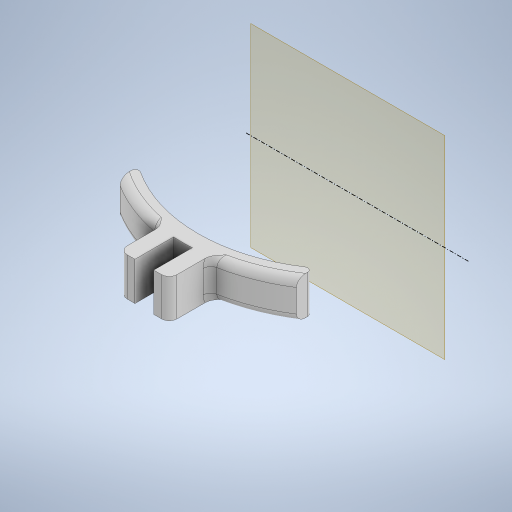
# Autodesk Inventor part: 날개꼽는파트
Saved by Autodesk Inventor 2023 (Build 270158000, 158)
## iProperties
Created: 2023-08-28
Part Number: 날개꼽는파트
Material: 일반
Document SubType Name: Modeling
Designer: rlatk
Density: 1 g/cm^3
Appearance: 기본값
Author: rlatk
Autodesk Inventor part; units mm, degrees
ref_plane "YZ Plane" through (0, 0, 0) normal (1, 0, 0) x (0, 1, 0)
ref_plane "XZ Plane" through (0, 0, 0) normal (0, 1, 0) x (-1, 0, 0)
sketch "스케치1" plane through (0, 0, 0) normal (0, 1, 0) x (-1, 0, 0)
  line L0 (-6.5, -10) -> (-6.5, 10)
  line L1 (6.5, 10) -> (6.5, -10)
  line L2 (6.5, -10) -> (-6.5, 10) construction
  line L3 (-6.5, -10) -> (6.5, 10) construction
  line L4 (2.45, -10) -> (-2.45, -10)
  line L5 (-2.45, -10) -> (-2.45, 10)
  line L6 (-2.45, 10) -> (2.45, 10)
  line L7 (2.45, 10) -> (2.45, -10)
  line L8 (2.45, -10) -> (-2.45, 10) construction
  line L9 (-2.45, -10) -> (2.45, 10) construction
  arc A0 (22.9827, -6.6573) -> (-22.9827, -6.6573) centre (0, -43) ccw
  arc A1 (22.9827, -11.4914) -> (-22.9827, -11.4914) centre (0, -43) ccw
  line L10 (22.9827, -11.4914) -> (22.9827, -6.6573)
  line L11 (-22.9827, -11.4914) -> (-22.9827, -6.6573)
  line L12 (-6.5, 10) -> (-2.45, 10)
  line L13 (2.45, 10) -> (6.5, 10)
  line L14 (6.5, -10) -> (2.45, -10)
  line L15 (-2.45, -10) -> (-6.5, -10)
  point P0 (0, 0)
  point P1 (6.5, -0.4941)
  point P2 (2.45, -0.0699)
  point P3 (-2.45, -0.0699)
  point P4 (-6.5, -0.4941)
  dimension "d0" = 13
  dimension "d1" = 20
  dimension "d2" = 4.9
  dimension "d3" = 86
  dimension "d4" = 4
  constraints: 32 end point, 8 parallel, 5 point on circle, 4 midpoint, 3 horizontal, 3 perpendicular, 2 centre point, 1 vertical
  measures "d0" distance of L0.end L1.start
  measures "d1" distance of L0.start L0.end
  measures "d2" distance of L5.end L6.end
  measures "d3" diameter of A0
  measures "d4" radial gap between concentric circles of A0 A1
sketch "스케치2" plane through (0, 0, 0) normal (0, 0, 1) x (1, 0, 0)
  point P0 (0, 0)
ref_plane "작업 평면1" through (0, 0, -43) normal (0, 0, 1) x (1, 0, 0)
sketch "스케치3" plane through (0, 0, -43) normal (0, 0, 1) x (1, 0, 0)
  line L0 (0, 0) -> (-26.5437, 0)
  line L1 (-26.5437, 0) -> (31.7273, 0)
  constraints: 4 end point, 1 horizontal, 1 point on line
extrude "돌출1" add sketch "스케치1" along normal blind 10 contours A1 L11 A0 L0 | L0 A0 L5 A1 | L0 L12 L5 A0 | L5 A0 L7 A1 | L7 A0 L1 A1 | L7 L13 L1 A0 | L1 A0 L10 A1
fillet "모깎기2" radius 1 2 edges at (22.9827, 5, -11.4914) (-22.9827, 5, -11.4914)
fillet "모깎기3" radius 2 6 edges at (-15.06, 0, -2.7235) (15.06, 0, -2.7235) (15.06, 10, -2.7235) (-15.06, 10, -2.7235) (6.5, 5, 10) (-6.5, 5, 10)
fillet "모깎기4" radius 2 2 edges at (-6.5, 5, -0.4941) (6.5, 5, -0.4941)
